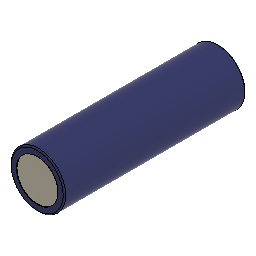
battery bank (Autodesk Fusion 360 archive; units mm, degrees)
design "27100 Battery"
Autodesk Fusion 360 part; units mm, degrees
sketch "Sketch1" plane through (0, 0, 0) normal (0, 1, 0) x (1, 0, 0)
  circle A0 centre (0, 0) radius 10.5
  dimension "d1" = 21
  constraint coincident A0.centre origin
  measures "d1" diameter of A0
extrude "Extrude2" add sketch "Sketch1" along normal blind 70
sketch "Sketch2" plane through (0, 0, 0) normal (0, -1, 0) x (1, 0, 0)
sketch "Sketch3" plane through (0, 0, 0) normal (0, -1, 0) x (1, 0, 0)
  circle A0 centre (0, 0) radius 10.5
  circle A1 centre (0, 0) radius 8
  dimension "d6" = 16
  constraint coincident A0.centre A1.centre
  measures "d6" diameter of A1
extrude "Extrude3" cut sketch "Sketch3" against normal blind 0.2 contours A1
sketch "Sketch4" plane through (0, 70, 0) normal (0, 1, 0) x (-1, 0, 0)
  circle A0 centre (0, 0) radius 10.5
  circle A1 centre (0, 0) radius 8
  circle A2 centre (0, 0) radius 7
  dimension "d9" = 16
  dimension "d10" = 14
  constraint concentric A0 A1
  constraint concentric A1 A2
  measures "d9" diameter of A1
  measures "d10" diameter of A2
extrude "Extrude4" cut sketch "Sketch4" against normal blind 3 contours A1
chamfer "Chamfer1" distance 0.5 distance2 3 1 edges at (6.5263, 70, -2.5313) measured on face at (1.3656, 70, -1.5351)
fillet "Fillet1" radius 0.5 1 edges at (-9.7894, 70, 3.797)
fillet "Fillet2" radius 0.5 1 edges at (-9.7894, 0, 3.797)
named bodies: "21700 battery"
